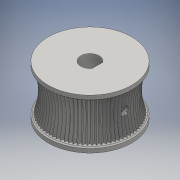
# Autodesk Inventor part: Roller
Saved by Autodesk Inventor 2016 (Build 200138000, 138)
## iProperties
Created: 2018-02-27
Part Number: Roller
Material: Generic
Document SubType Name: Modeling
Designer: Simon
Density: 1 g/cm^3
Appearance: Default
Author: Simon
Autodesk Inventor part; units mm, degrees
sketch "Sketch1" plane through (0, 0, 0) normal (0, 0, 1) x (1, 0, 0)
  circle A0 centre (0, 0) radius 12.5
  dimension "d0" = 25
  constraints: 1 centre point, 1 coincident
  measures "d0" diameter of A0
extrude "Extrusion1" add sketch "Sketch1" along normal blind 15
sketch "Sketch2" plane through (0, 0, 15) normal (0, 0, 1) x (1, 0, 0)
  circle A0 centre (0, 0) radius 12.5 projected
  point P0 (0, -12.5)
  constraints: 1 vertical alignment, 1 other
ref_plane "Work Plane2" through (0, 0, 15) normal (0, -1, 0) x (1, 0, 0)
ref_plane "Work Plane1" through (0, -12.5, 15) normal (0, -1, 0) x (1, 0, 0)
sketch "Sketch3" plane through (0, 0, 15) normal (0, -1, 0) x (1, 0, 0)
  line L0 (-12.5, -15) -> (-12.5, 0) projected
  line L1 (-12.5, -15) -> (12.5, -15) projected
  line L2 (-12.5, 0) -> (-12.5, -15)
  arc A0 (-12.5, -15) -> (-12.5, 0) centre (-31.0405, -7.5) ccw
  line L3 (0, -18) -> (0, 3) projected
  point P0 (0, -15)
  dimension "d4" = 20
  constraints: 2 end point, 2 point on circle, 1 centre point, 1 point on line, 1 vertical
  measures "d4" radius of A0
revolve "Revolution1" cut sketch "Sketch3" angle 360 about axis through (0, 0, -10) along (0, 0, 1)
ref_plane "Work Plane3" through (0, 0, 13.5) normal (0, 0, 1) x (1, 0, 0)
sketch "Sketch4" plane through (0, 0, 13.5) normal (0, 0, 1) x (1, 0, 0)
  arc A0 (0, 12.022) -> (-1.1414, 11.9677) centre (0, 0) ccw
  line L0 (0, 12.022) -> (-0.5864, 11.0064)
  line L1 (0, 12.022) -> (1.1727, 12.022) construction
  line L2 (-0.5864, 11.0064) -> (-1.1414, 11.9677)
  line L3 (-0.5864, 11.0064) -> (0.5237, 11.0064) construction
  dimension "d8" = 120
  dimension "d9" = 120
  constraints: 8 end point, 2 equal length, 2 horizontal, 2 point on circle, 1 centre point, 1 coincident
  measures "d8" angle of L0 L1
  measures "d9" angle of L3 L2
sketch "Sketch5" plane through (0, 0, 0) normal (1, 0, 0) x (0, 1, 0)
  arc A0 (12.5, 15) -> (12.5, 0) centre (31.0405, 7.5) ccw projected
  arc A1 (12.0986, 13.9192) -> (12.0986, 1.0808) centre (31.0405, 7.5) ccw
  line L0 (12.0986, 13.9192) -> (12.0986, 1.0808) construction
  line L1 (12.0986, 13.9192) -> (24.937, 13.9192) construction
  point P0 (0, 0)
  dimension "d10" = 90
  constraints: 4 end point, 4 point on circle, 1 centre point, 1 horizontal, 1 perpendicular
  measures "d10" angle of L0 L1
sweep "Sweep1" cut profiles "Sketch4" path "Sketch5" path curves A0
pattern_circular "Circular Pattern1" count 73 over 360 about axis through (0, 0, -10) along (0, 0, 1) of "Sweep1"
sketch "Sketch6" plane through (0, 0, 15) normal (0, 0, 1) x (1, 0, 0)
  circle A0 centre (0, 0) radius 12.5
  dimension "d16" = 25
  constraints: 1 centre point, 1 coincident
  measures "d16" diameter of A0
extrude "Extrusion2" add sketch "Sketch6" against normal blind 1.5
sketch "Sketch7" plane through (0, 0, 0) normal (0, 0, -1) x (-1, 0, 0)
  circle A0 centre (0, 0) radius 12.5
  dimension "d19" = 25
  constraints: 1 centre point, 1 coincident
  measures "d19" diameter of A0
extrude "Extrusion3" add sketch "Sketch7" against normal blind 1.5
chamfer "Chamfer1" distance 0.3 angle 45 2 edges at (-12.5, 0, 13.5) (12.5, 0, 1.5)
sketch "Sketch8" plane through (0, 0, 15) normal (0, 0, 1) x (1, 0, 0)
  arc A0 (2.25, 1.5811) -> (2.25, -1.5811) centre (0, 0) ccw
  line L0 (2.25, 1.5811) -> (2.25, -1.5811)
  dimension "d25" = 5.5
  dimension "d26" = 0.5
  constraints: 2 end point, 2 point on circle, 1 centre point, 1 coincident, 1 vertical
  measures "d25" diameter of A0
  measures "d26" distance edge to line of A0 L0
extrude "Extrusion4" cut sketch "Sketch8" against normal through all
sketch "Sketch9" plane through (2.25, -1.5811, 15) normal (-1, 0, 0) x (0, 0, 1)
  circle A0 centre (-7.5, 1.4318) radius 1
  point P0 (-15, 1.5811)
  dimension "d29" = 2
  constraints: 1 centre point
  measures "d29" diameter of A0
extrude "Extrusion5" cut sketch "Sketch9" against normal through all
ref_plane "Work Plane4" through (15.25, 0, 0) normal (1, 0, 0) x (0, 1, 0)
sketch "Sketch11" plane through (15.25, 0, 0) normal (1, 0, 0) x (0, 1, 0)
  circle A0 centre (-0.1493, 7.5) radius 1.25
  point P0 (0, 0)
  dimension "d34" = 2.5
  constraints: 1 centre point, 1 coincident
  measures "d34" diameter of A0
extrude "Extrusion6" cut sketch "Sketch11" against normal blind 6
body "Solid1"
